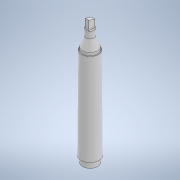
# Autodesk Inventor part: MARCADOR
Saved by Autodesk Inventor 2022 (Build 260153000, 153)
## iProperties
Created: 2022-09-01
Part Number: MARCADOR
Material: Genérico
Document SubType Name: Modeling
Designer: Usuario
Density: 1 g/cm^3
Appearance: Valor por defecto
Author: Usuario
Autodesk Inventor part; units mm, degrees
ref_plane "YZ Plane" through (0, 0, 0) normal (1, 0, 0) x (0, 1, 0)
sketch "Boceto1" plane through (0, 0, 0) normal (0, 1, 0) x (-1, 0, 0)
  circle A0 centre (0, 0) radius 7.275
  circle A1 centre (0, 0) radius 8.7
  dimension "d0" = 14.55
  dimension "d1" = 17.4
  constraints: 2 centre point, 2 coincident
  measures "d0" diameter of A0
  measures "d1" diameter of A1
extrude "Extrusión1" add sketch "Boceto1" along normal blind 5.9 contours A0
sketch "Boceto2" plane through (0, 5.9, 0) normal (0, 1, 0) x (1, 0, 0)
  circle A0 centre (0, 0) radius 8.7
  dimension "d5" = 17.4
  constraints: 1 centre point
  measures "d5" diameter of A0
ref_plane "Plano de trabajo1" through (0, 95.1, 0) normal (0, -1, 0) x (1, 0, 0)
sketch "Boceto3" plane through (0, 95.1, 0) normal (0, -1, 0) x (1, 0, 0)
  circle A0 centre (0, 0) radius 8.115
  dimension "d7" = 16.23
  constraints: 1 centre point, 1 coincident
  measures "d7" diameter of A0
loft "Solevación1" add profiles "Boceto3", "Boceto2"
sketch "Boceto4" plane through (0, 0, 0) normal (0, -1, 0) x (1, 0, 0)
  circle A0 centre (0, 0) radius 7.275
  circle A1 centre (0, 0) radius 6.515
  dimension "d12" = 13.03
  constraints: 2 centre point, 2 coincident
  measures "d12" diameter of A1
extrude "Extrusión2" cut sketch "Boceto4" against normal blind 1.08 contours A1
sketch "Boceto5" plane through (0, 95.1, 0) normal (0, 1, 0) x (1, 0, 0)
  circle A0 centre (0, 0) radius 7.21
  dimension "d15" = 14.42
  constraints: 1 centre point, 1 coincident
  measures "d15" diameter of A0
extrude "Extrusión3" add sketch "Boceto5" along normal blind 2.65
ref_plane "Plano de trabajo2" through (0, 106.9, 0) normal (0, 1, 0) x (1, 0, 0)
sketch "Boceto6" plane through (0, 106.9, 0) normal (0, 1, 0) x (1, 0, 0)
  circle A0 centre (0, 0) radius 3.95
  dimension "d19" = 7.9
  constraints: 1 centre point, 1 coincident
  measures "d19" diameter of A0
loft "Solevación2" add profiles "Boceto6" section 2 edges at (-7.21, 97.75, 0)
sketch "Boceto7" plane through (0, 106.9, 0) normal (0, 1, 0) x (1, 0, 0)
  circle A0 centre (0, 0) radius 3.95
  constraints: 1 centre point, 1 coincident
extrude "Extrusión4" add sketch "Boceto7" along normal blind 6.58
sketch "Boceto8" plane through (0, 113.48, 0) normal (0, 1, 0) x (1, 0, 0)
  line L0 (1.8, 2.78) -> (-1.8, 2.78)
  line L1 (-1.8, 2.78) -> (-1.8, -2.78)
  line L2 (-1.8, -2.78) -> (1.8, -2.78)
  line L3 (1.8, -2.78) -> (1.8, 2.78)
  circle A0 centre (0, 0) radius 3.95 projected
  line L4 (1.8, 2.78) -> (-1.8, -2.78) construction
  line L5 (-1.8, 2.78) -> (1.8, -2.78) construction
  dimension "d26" = 3.6
  dimension "d27" = 5.56
  constraints: 12 end point, 2 midpoint, 2 parallel, 1 horizontal, 1 perpendicular
  measures "d26" distance of L2.end L1.end
  measures "d27" distance of L1.end L0.end
extrude "Extrusión5" add sketch "Boceto8" along normal blind 8.65 contours L3 L2 L1 L0
sketch "Boceto9" plane through (-1.8, 113.48, -2.78) normal (-1, 0, 0) x (0, 0, 1)
  line L0 (0, 0) -> (0, 8.65) projected
  line L1 (0, 0) -> (0, 7)
  line L2 (0, 8.65) -> (5.56, 8.65) projected
  line L3 (0, 7) -> (5.56, 8.65)
  point P0 (2.78, -113.48)
  dimension "d30" = 7
  constraints: 4 end point, 1 point on line
  measures "d30" distance of L0.start L1.end
extrude "Extrusión6" cut sketch "Boceto9" against normal blind 8.65
